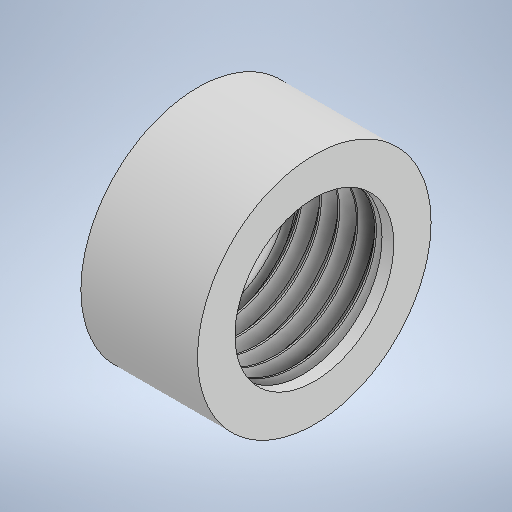
# Autodesk Inventor part: Innerer Differential Wurm Getriebe
Saved by Autodesk Inventor 2025 (Build 290162010, 162A)
## iProperties
Created: 2024-11-22
Part Number: Innerer Differential Wurm Getriebe
Material: Generisch
Document SubType Name: Modeling
Designer: jensb
Density: 1 g/cm^3
Appearance: Vorgabe
Author: jensb
Autodesk Inventor part; units mm, degrees
ref_plane "YZ Plane" through (0, 0, 0) normal (1, 0, 0) x (0, 1, 0)
ref_plane "XZ Plane" through (0, 0, 0) normal (0, 1, 0) x (-1, 0, 0)
ref_plane "XY Plane" through (0, 0, 0) normal (0, 0, 1) x (1, 0, 0)
sketch "Skizze1" plane through (0, 0, 0) normal (0, 0, 1) x (1, 0, 0)
  line L0 (-25, 0) -> (25, 0)
  line L1 (-25, 34) -> (25, 34)
  line L2 (-25, 34) -> (-25, 50)
  line L3 (-25, 50) -> (25, 50)
  line L4 (25, 50) -> (25, 34)
  point P0 (0, 0)
  point P1 (0, 0)
  dimension "d0" = 68
  dimension "d1" = 100
  dimension "d2" = 50
  constraints: 10 end point, 2 horizontal, 2 perpendicular, 2 vertical alignment, 1 coincident, 1 midpoint, 1 vertical
  measures "d0" diameter of L1 L0
  measures "d1" diameter of L3 L0
  measures "d2" distance between parallel lines of L4 L2
revolve "Umdrehung1" add sketch "Skizze1" angle 360 about axis through (-25, 0, 0) along (1, 0, 0)
sketch "Skizze2" plane through (0, 0, 0) normal (0, 0, 1) x (1, 0, 0)
  arc A0 (23.9, -39.278) -> (26.1, -39.278) centre (25, -11.75) ccw
  line L0 (25, -23.5023) -> (25, -32.75) construction
  line L1 (25, -34) -> (25, 34) projected
  line L2 (27.65, -32.75) -> (22.35, -32.75) construction
  line L3 (25, -34) -> (-25, -34) projected
  line L4 (25, -34) -> (-25, -34) projected
  line L5 (23.9, -39.278) -> (21.4388, -34)
  line L6 (26.1, -39.278) -> (28.5612, -34)
  line L7 (28.5612, -34) -> (21.4388, -34)
  point P0 (0, 0)
  point P1 (25, 0)
  dimension "d4" = 27.55
  dimension "d5" = 2.2
  dimension "d9" = 11.75
  dimension "d10" = 21
  dimension "d11" = 5.3
  dimension "d21" = 25
  constraints: 10 end point, 3 vertical alignment, 2 point on circle, 1 centre point, 1 collinear, 1 horizontal, 1 horizontal alignment, 1 midpoint, 1 point on line, 1 vertical, 1 other
  measures "d4" radius of A0
  measures "d5" distance of L6.start L5.start
  measures "d9" vertical distance of point (0, 0) A0.centre
  measures "d10" distance from line of A0.centre L2
  measures "d11" distance of L2.start L2.end
  measures "d21" angle of L1 L5
coil "Spirale1" sketch "Skizze2" operation cut axis through (-10, 0, 0) along (-1, 0, 0) pitch 7.85 turns 5.732484 hand right
sketch "Skizze3" plane through (-25, 0, 0) normal (-1, 0, 0) x (0, 0, 1)
  circle A0 centre (0, 0) radius 50 projected
  circle A1 centre (0, 0) radius 50
  circle A2 centre (0, 0) radius 34
  point P0 (0, 0)
  constraints: 2 centre point, 2 coincident
extrude "Extrusion1" add sketch "Skizze3" against normal blind 5
sketch "Skizze4" plane through (25, 0, 0) normal (1, 0, 0) x (0, 0, -1)
  circle A0 centre (0, 0) radius 50
  circle A1 centre (0, 0) radius 34
  constraints: 2 centre point, 2 coincident
extrude "Extrusion2" add sketch "Skizze4" against normal blind 5
